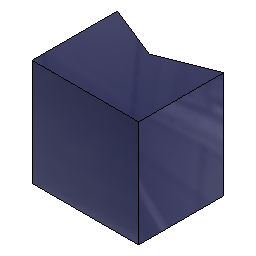
control electronics v5 (Autodesk Fusion 360 design; units mm, degrees)
Autodesk Fusion 360 part; units mm, degrees
sketch "Sketch1" plane through (0, 0, 0) normal (0, 0, 1) x (1, 0, 0)
  line L0 (0, 0) -> (2.5, 0)
  line L1 (2.5, 0) -> (2.5, 2)
  line L2 (0, 2) -> (0, 0)
  line L3 (0, 2) -> (1.25, 1.5011)
  line L4 (1.25, 1.5011) -> (2.5, 2)
  dimension "d4" = 2
  dimension "d5" = 1.3459
  dimension "d6" = 1.3459
  dimension "d7" = 1.5011
  dimension "d8" = 2.5
  constraint horizontal L0
  constraint vertical L1
  constraint vertical L2
  constraint coincident L0.start L2.end
  measures "d4" distance of L0.end L1.end
  measures "d5" distance of L2.start L3.end
  measures "d6" distance of L1.end L3.end
  measures "d7" distance of L0 L3.end
  measures "d8" distance of L0.start L0.end
extrude "Extrude1" add sketch "Sketch1" along normal blind 2.5
